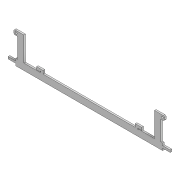
# Autodesk Inventor part: rod_2
Saved by Autodesk Inventor 2022 (Build 260153000, 153)
## iProperties
Created: 2023-04-07
Part Number: rod_2
Material: 一般
Document SubType Name: Modeling
Designer: may9c
Density: 79.16 g/cm^3
Appearance: 預設
Mass: 822.393 g
Surface Area: 88.4 cm^2
Volume: 10.389 cm^3
Author: may9c
Autodesk Inventor part; units mm, degrees
ref_plane "YZ Plane" through (0, 0, 0) normal (1, 0, 0) x (0, 1, 0)
ref_plane "XY Plane" through (0, 0, 0) normal (0, 0, 1) x (1, 0, 0)
sketch "草圖1" plane through (0, 0, 0) normal (0, 0, 1) x (1, 0, 0)
  line L0 (0, 6) -> (0, -6)
  line L1 (0, -6) -> (-136, -6)
  line L2 (-136, -6) -> (-136, 6)
  line L3 (-150, 2) -> (-136, 2)
  line L4 (-136, 2) -> (-136, -2)
  line L5 (-136, -2) -> (-150, -2)
  line L6 (-150, -2) -> (-150, 2)
  line L7 (-210, 0) -> (210, 0) projected
  line L8 (0, -17.4828) -> (0, 62.8971) projected
  line L9 (0, -6) -> (136, -6)
  line L10 (136, -6) -> (136, 6)
  line L11 (150, 2) -> (136, 2)
  line L12 (136, -2) -> (150, -2)
  line L13 (150, -2) -> (150, 2)
  line L14 (136, -6) -> (136, -2)
  line L15 (145, 2) -> (139, 2)
  line L16 (-97.5, 7) -> (-97.5, 12)
  line L17 (-91, 7) -> (-97.5, 7)
  line L18 (97.5, 7) -> (97.5, 12)
  line L19 (97.5, 12) -> (87.5, 12)
  line L20 (90, 7) -> (97.5, 7)
  line L21 (90, 7) -> (90, 5)
  line L22 (90, 5) -> (91, 5)
  line L23 (91, 5) -> (91, 6)
  line L24 (-136, 6) -> (-91, 6)
  line L25 (-85.5, 6) -> (85.5, 6)
  line L26 (91, 6) -> (136, 6)
  line L27 (-85.5, 12) -> (-85.5, 6)
  line L28 (87.5, 12) -> (85.5, 12)
  line L29 (85.5, 12) -> (85.5, 6)
  line L30 (-97.5, 12) -> (-85.5, 12)
  line L31 (-91, 7) -> (-91, 8)
  line L32 (-91, 8) -> (-90, 8)
  line L33 (-90, 8) -> (-90, 7)
  line L34 (-90, 7) -> (-90, 6)
  line L35 (-91, 6) -> (-90, 6)
  point P0 (0, 0)
  point P1 (-136, 2)
  point P2 (136, -6)
  point P3 (136, -2)
  dimension "d2" = 4
  dimension "d14" = 2
  dimension "d17" = 12
  dimension "d57" = 14
  dimension "d58" = 300
  dimension "d62" = 2
  dimension "d63" = 85.5
  dimension "d64" = 85.5
  dimension "d65" = 12
  dimension "d66" = 5
  dimension "d67" = 6
  dimension "d68" = 6.5
  dimension "d69" = 136
  dimension "d70" = 14
  dimension "d71" = 136
  dimension "d72" = 272
  constraints: 68 end point, 10 horizontal, 10 symmetric about line, 5 perpendicular, 3 parallel, 3 point on line, 1 collinear, 1 vertical, 1 other
  measures "d2" distance between parallel lines of L5 L3
  measures "d14" distance of L19.end L28.end
  measures "d17" distance between parallel lines of L1 L24
  measures "d57" distance between parallel lines of L13 L10
  measures "d58" distance between parallel lines of L13 L6
  measures "d62" distance of L24.end L31.end
  measures "d63" distance between parallel lines of L0 L27
  measures "d64" distance between parallel lines of L29 L0
  measures "d65" distance between parallel lines of L27 L16
  measures "d66" distance between parallel lines of L30 L17
  measures "d67" distance between parallel lines of L25 L30
  measures "d68" distance of L17.start L16.start
  measures "d69" distance between parallel lines of L10 L0
  measures "d70" distance between parallel lines of L2 L6
  measures "d71" distance of L0.end L1.end
  measures "d72" distance between parallel lines of L10 L2
extrude "擠出1" add sketch "草圖1" along normal blind 3
ref_plane "工作平面1" through (0, 0, 1.5) normal (0, 0, 1) x (1, 0, 0)
sketch "草圖7" plane through (0, 0, 0) normal (0, 0, -1) x (-1, 0, 0)
  line L0 (-210, 0) -> (210, 0) projected
  circle A0 centre (129.5, 0) radius 12.5
  line L1 (150, -2) -> (136, -2) projected
  line L2 (142, -2) -> (142, 2)
  line L3 (136, 2) -> (150, 2) projected
  line L4 (150, 2) -> (150, -2) projected
  circle A1 centre (129.5, 0) radius 2.05
  line L5 (136, 6) -> (136, 2) projected
  point P0 (0, 0)
  dimension "d36" = 25
  dimension "d38" = 4.1
  dimension "d73" = 6
  constraints: 2 centre point, 2 end point, 2 point on line, 1 coincident, 1 tangent, 1 vertical
  measures "d36" diameter of A0
  measures "d38" diameter of A1
  measures "d73" distance between parallel lines of L2 L5
extrude "擠出5" cut sketch "草圖7" against normal up to surface (3 mm away) contours A1 L0 | L0 A1
sketch "草圖8" plane through (0, 0, 3) normal (0, 0, 1) x (1, 0, 0)
  line L0 (-90, 6) -> (-136, 6) projected
  line L1 (-133, 6) -> (-121, 6)
  line L2 (-121, 6) -> (-121, 51)
  line L3 (-121, 51) -> (-136, 51)
  line L4 (-133, 43) -> (-133, 6)
  line L5 (-136, 6) -> (-136, 2) projected
  line L6 (-136, 51) -> (-139.5, 51)
  line L7 (-139.5, 51) -> (-139.5, 43)
  line L8 (-139.5, 43) -> (-133, 43)
  circle A0 centre (-135.5, 47) radius 2.05
  circle A1 centre (-129.5, 0) radius 2.05 projected
  circle A2 centre (-135.5, 47) radius 6.5 construction
  line L9 (-136, 2) -> (-150, 2) projected
  line L10 (-150, 2) -> (-150, 58.0765) construction
  line L11 (-150, 58.0765) -> (-142, 58.0765) construction
  line L12 (-142, 58.0765) -> (-142, 42.2693) construction
  line L13 (-137.3204, 6) -> (-133, 6)
  line L14 (-133, 6) -> (-133, 16.271)
  circle A3 centre (-129.5, 16.6771) radius 2.05
  circle A4 centre (-129.5, 16.6771) radius 12.5 construction
  point P0 (0, 0)
  point P1 (-91, 6)
  dimension "d55" = 25
  dimension "d41" = 3
  dimension "d42" = 15
  dimension "d43" = 45
  dimension "d45" = 8
  dimension "d50" = 13
  dimension "d51" = 47
  dimension "d52" = 6.5
  dimension "d74" = 6
  constraints: 24 end point, 5 perpendicular, 3 centre point, 3 horizontal, 3 parallel, 3 point on line, 2 coincident, 2 equal radius, 1 tangent, 1 vertical, 1 vertical alignment, 3 other
  measures "d41" distance between parallel lines of L5 L4
  measures "d42" distance of L2.end L3.end
  measures "d43" distance between parallel lines of L0 L3
  measures "d45" distance between parallel lines of L8 L6
  measures "d50" diameter of A2
  measures "d51" vertical distance of A1.centre A0.centre
  measures "d52" distance between parallel lines of L4 L7
  measures "d74" distance between parallel lines of L5 L12
extrude "擠出6" add sketch "草圖8" against normal up to surface (3 mm away) contours L0 L4 L8 L7 L6 L3 L2 | A1 | A3
fillet "圓角2" radius 2 2 edges at (-139.5, 51, 1.5) (-139.5, 43, 1.5)
mirror "鏡射6" about plane through (0, 0, 0) normal (1, 0, 0) of "擠出5", "擠出6", "圓角2"
